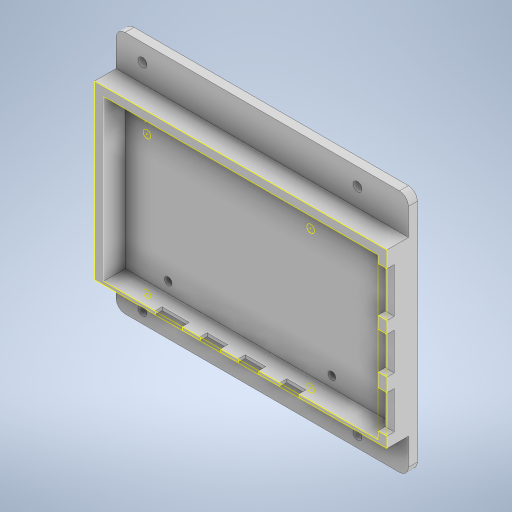
# Autodesk Inventor part: RPIcaseBottom
Saved by Autodesk Inventor 2024 (Build 280153000, 153)
## iProperties
Created: 2023-07-18
Part Number: RPIcaseBottom
Material: Generic
Document SubType Name: Modeling
Designer: 18179
Density: 1 g/cm^3
Appearance: Default
Autodesk Inventor part; units mm, degrees
ref_plane "YZ Plane" through (0, 0, 0) normal (1, 0, 0) x (0, 1, 0)
ref_plane "XZ Plane" through (0, 0, 0) normal (0, 1, 0) x (-1, 0, 0)
ref_plane "XY Plane" through (0, 0, 0) normal (0, 0, 1) x (1, 0, 0)
sketch "0" plane through (0, 0, 0) normal (0, 0, 1) x (1, 0, 0)
  line L0 (79, 0) -> (0, 0)
  arc A0 (0, 0) -> (-3, -3) centre (0, -3) ccw
  line L1 (-3, -3) -> (-3, -53)
  arc A1 (-3, -53) -> (0, -56) centre (0, -53) ccw
  line L2 (0, -56) -> (79, -56)
  arc A2 (79, -56) -> (82, -53) centre (79, -53) ccw
  line L3 (82, -53) -> (82, -3)
  arc A3 (82, -3) -> (79, 0) centre (79, -3) ccw
  circle A4 centre (0.5, -3.5) radius 1.35
  circle A5 centre (0.5, -52.5) radius 1.35
  line L4 (3.73, -49.89) -> (3.73, -57.5)
  line L5 (12.67, -57.5) -> (12.67, -49.89)
  line L6 (5.03, -57.5) -> (11.37, -57.5)
  line L7 (19.75, -50.3) -> (19.75, -57.8)
  line L8 (26.25, -57.8) -> (26.25, -50.3)
  line L9 (20.2, -57.8) -> (25.8, -57.8)
  line L10 (33.25, -50.3) -> (33.25, -57.8)
  line L11 (39.75, -57.8) -> (39.75, -50.3)
  line L12 (33.7, -57.8) -> (39.3, -57.8)
  line L13 (54, -55.9) -> (54, -58.1)
  line L14 (48, -55.9) -> (48, -58.1)
  line L15 (48.3, -58.4) -> (53.7, -58.4)
  line L16 (68.53, -53.65) -> (85, -53.65)
  line L17 (85, -53.35) -> (85, -40.65)
  line L18 (85, -40.35) -> (68.53, -40.35)
  line L19 (68.44, -22.45) -> (85, -22.45)
  line L20 (85.6, -23.75) -> (85.6, -34.25)
  line L21 (68.44, -35.55) -> (85, -35.55)
  line L22 (84.8, -2.3) -> (63.85, -2.3)
  line L23 (85, -18) -> (85, -2.5)
  line L24 (63.85, -18.2) -> (84.8, -18.2)
  circle A6 centre (58.5, -3.5) radius 1.35
  circle A7 centre (58.5, -52.5) radius 1.35
  line L25 (3.73, -57.5) -> (12.67, -57.5)
  line L26 (19.75, -57.8) -> (26.25, -57.8)
  line L27 (33.25, -57.8) -> (39.75, -57.8)
  line L28 (54, -58.1) -> (53.7, -58.4)
  line L29 (48.3, -58.4) -> (48, -58.1)
  line L30 (85, -53.65) -> (85, -40.35)
  line L31 (85, -35.55) -> (85.6, -35.55)
  line L32 (85.6, -35.55) -> (85.6, -22.45)
  line L33 (85.6, -22.45) -> (85, -22.45)
  line L34 (84.8, -18.2) -> (85, -18.2)
  line L35 (85, -18.2) -> (85, -2.3)
  line L36 (85, -2.3) -> (84.8, -2.3)
  line L37 (84.8, -2.3) -> (84.8, -18.2)
  line L38 (-3, -28) -> (-18, -28)
  line L39 (3.73, -57.5) -> (-18, -57.5)
  line L40 (-18, -57.5) -> (85.6, -57.5)
  line L41 (79, 0.3263) -> (0, 0.3263)
  line L42 (39.5, 0.3263) -> (39.5, 3.5013)
  line L43 (0, -56.3549) -> (79, -56.3549)
  line L44 (3.4071, -49.89) -> (3.4071, -57.5)
  line L45 (13.029, -49.89) -> (13.029, -57.859)
  line L46 (13.029, -57.859) -> (3.73, -57.859)
  line L47 (19.369, -50.3) -> (19.369, -58.181)
  line L48 (19.369, -58.181) -> (26.631, -58.181)
  line L49 (26.631, -58.181) -> (26.631, -50.3)
  line L50 (32.869, -50.3) -> (32.869, -58.181)
  line L51 (32.869, -58.181) -> (40.131, -58.181)
  line L52 (40.131, -58.181) -> (40.131, -50.3)
  line L53 (47.619, -55.9) -> (47.619, -58.2578)
  line L54 (47.619, -58.2578) -> (48.1422, -58.781)
  line L55 (48.1422, -58.781) -> (53.8578, -58.781)
  line L56 (53.8578, -58.781) -> (54.381, -58.2578)
  line L57 (54.381, -58.2578) -> (54.381, -55.9)
  line L58 (82.381, -53) -> (82.381, -3)
  line L59 (-3.381, -3) -> (-3.381, -53)
  line L60 (-18, -57.5) -> (39.5, -57.5)
  line L61 (39.5, -57.5) -> (39.5, 3.5013) construction
  line L62 (39.5, 3.5013) -> (-18, 3.5013)
  line L63 (-18, 3.5013) -> (-18, -57.5)
  line L64 (39.5, 3.5013) -> (85.6, 3.5013)
  line L65 (85.6, 3.5013) -> (85.6, -57.5)
  line L66 (85.6, -57.5) -> (39.5, -57.5)
  line L67 (39.5, -57.5) -> (39.5, 3.5013) construction
  line L68 (-3.381, -3) -> (0, -3)
  line L69 (0, -3) -> (0, 0.3263)
  line L70 (0, 0.3263) -> (-3.381, 0.3263)
  line L71 (-3.381, 0.3263) -> (-3.381, -3)
  line L72 (79, 0.3263) -> (82.381, 0.3263)
  line L73 (82.381, 0.3263) -> (82.381, -3)
  line L74 (82.381, -3) -> (79, -3)
  line L75 (79, -3) -> (79, 0.3263)
  line L76 (79, -56.3549) -> (82.381, -56.3549)
  line L77 (82.381, -56.3549) -> (82.381, -53)
  line L78 (82.381, -53) -> (79, -53)
  line L79 (79, -53) -> (79, -56.3549)
  line L80 (-3.381, -53) -> (0, -53)
  line L81 (0, -53) -> (0, -56.3549)
  line L82 (0, -56.3549) -> (-3.381, -56.3549)
  line L83 (-3.381, -56.3549) -> (-3.381, -53)
  line L84 (85, -53.65) -> (85.6, -53.65)
  line L85 (85.6, -53.65) -> (85.6, -40.35)
  line L86 (85.6, -40.35) -> (85, -40.35)
  line L87 (85, -40.35) -> (85, -53.65)
  line L88 (85, -18.2) -> (85.6, -18.2)
  line L89 (85.6, -18.2) -> (85.6, -2.3)
  line L90 (85.6, -2.3) -> (85, -2.3)
  line L91 (85, -2.3) -> (85, -18.2)
  line L92 (-18, -28) -> (-14.825, -28)
  line L93 (-14.825, -28) -> (-3.381, -28)
  line L94 (-3.381, -28) -> (-3.381, 0.3263)
  line L95 (-3.381, 0.3263) -> (-14.825, 0.3263)
  line L96 (-14.825, 0.3263) -> (-14.825, -28)
  line L97 (-14.825, -28) -> (-3.381, -28)
  line L98 (-3.381, -28) -> (-3.381, -56.3549)
  line L99 (-3.381, -56.3549) -> (-14.825, -56.3549)
  line L100 (-14.825, -56.3549) -> (-14.825, -28)
  point P0 (19.369, -57.5)
  point P1 (19.369, -56.3549)
  point P2 (13.029, -56.3549)
  point P3 (13.029, -57.5)
  point P4 (32.869, -57.5)
  point P5 (32.869, -56.3549)
  point P6 (26.631, -56.3549)
  point P7 (26.631, -57.5)
  point P8 (47.619, -57.5)
  point P9 (47.619, -56.3549)
  point P10 (40.131, -56.3549)
  point P11 (40.131, -57.5)
  point P12 (54.381, -56.3549)
  point P13 (54.381, -57.5)
  point P14 (82.381, -53.65)
  point P15 (82.381, -35.55)
  point P16 (82.381, -40.35)
  point P17 (82.381, -18.2)
  point P18 (82.381, -22.45)
  point P19 (82.381, -2.3)
  point P20 (3.4071, -56.3549)
  dimension "d0" = 15
  dimension "d2" = 3.175
  dimension "d3" = 0.381
  dimension "d4" = 0.381
  dimension "d5" = 0.381
  dimension "d6" = 0.381
  dimension "d7" = 0.381
  dimension "d8" = 3.175
  constraints: 202 end point, 27 parallel, 16 perpendicular, 14 horizontal, 8 centre point, 8 point on circle, 5 point on line, 2 collinear, 2 midpoint, 2 vertical, 9 other
  measures "d0" distance of L38.start L38.end
  measures "d2" distance of L42.start L42.end
  measures "d3" distance between parallel lines of L7 L47
  measures "d4" distance between parallel lines of L10 L50
  measures "d5" distance between parallel lines of L29 L54
  measures "d6" distance between parallel lines of L3 L58
  measures "d7" distance between parallel lines of L1 L59
  measures "d8" distance of L38.end L92.end
extrude "Extrusion1" add sketch "0" along normal blind 7.62 contours L41 L42 L64 L65 L90 L36 L22 L73 L72 | L70 L95 L96 L38 L63 L62 L42 L41 | L69 L68 A4 | A4 L68 L69 | L24 L34 L88 L65 L33 L19 L58 | L80 L81 A5 | A5 L81 L80 | L100 L99 L82 L43 L44 L39 L63 L38 | L21 L31 L65 L86 L18 L58 | L16 L84 L65 L40 L57 L43 L76 L77 | L43 L47 L40 L45 | L43 L50 L40 L49 | L53 L40 L52 L43 | A6 | A7
sketch "Sketch3" plane through (0, 0, 0) normal (0, 0, -1) x (-1, 0, 0)
  line L0 (-85.6, 3.5013) -> (18, 3.5013) projected
  line L1 (-54.381, -57.5) -> (-85.6, -57.5) projected
  line L2 (18, 3.5013) -> (-85.6, 3.5013)
  line L3 (-85.6, 3.5013) -> (-85.6, -57.5)
  line L4 (-85.6, -57.5) -> (18, -57.5)
  line L5 (18, -57.5) -> (18, 3.5013)
  circle A0 centre (-0.5, -3.5) radius 1.35 projected
  circle A1 centre (-0.5, -52.5) radius 1.35 projected
  circle A2 centre (-58.5, -52.5) radius 1.35 projected
  circle A3 centre (-58.5, -3.5) radius 1.35 projected
  line L6 (18, -57.5) -> (-85.6, -57.5)
  line L7 (-85.6, -57.5) -> (-85.6, -67.025)
  line L8 (-82.425, -70.2) -> (14.825, -70.2)
  line L9 (18, -67.025) -> (18, -57.5)
  line L10 (18, 3.5013) -> (-85.6, 3.5013)
  line L11 (-85.6, 3.5013) -> (-85.6, 13.0263)
  line L12 (-82.425, 16.2013) -> (14.825, 16.2013)
  line L13 (18, 13.0263) -> (18, 3.5013)
  arc A4 (18, 13.0263) -> (14.825, 16.2013) centre (14.825, 13.0263) ccw
  arc A5 (-82.425, 16.2013) -> (-85.6, 13.0263) centre (-82.425, 13.0263) ccw
  line L14 (-0.5, -52.5) -> (-58.5, -3.5) construction
  line L15 (-58.5, -3.5) -> (-58.5, -52.5) construction
  line L16 (-58.5, -52.5) -> (-0.5, -3.5) construction
  arc A6 (14.825, -70.2) -> (18, -67.025) centre (14.825, -67.025) ccw
  arc A7 (-85.6, -67.025) -> (-82.425, -70.2) centre (-82.425, -67.025) ccw
  line L17 (-29.5, -28) -> (-29.5, -66.1) construction
  line L18 (-29.5, -66.1) -> (-29.5, 10.1) construction
  line L19 (-29.5, 10.1) -> (8.6, 10.1) construction
  line L20 (8.6, 10.1) -> (-67.6, 10.1) construction
  line L21 (-29.5, -66.1) -> (8.6, -66.1) construction
  line L22 (8.6, -66.1) -> (-67.6, -66.1) construction
  circle A8 centre (8.6, -66.1) radius 1.5875
  circle A9 centre (-67.6, -66.1) radius 1.5875
  circle A10 centre (-67.6, 10.1) radius 1.5875
  circle A11 centre (8.6, 10.1) radius 1.5875
  point P0 (0, 0)
  point P1 (-85.6, -70.2)
  point P2 (-85.6, 16.2013)
  dimension "d11" = 12.7
  dimension "d12" = 12.7
  dimension "d13" = 3.175
  dimension "d14" = 3.175
  dimension "d15" = 38.1
  dimension "d16" = 76.2
  dimension "d17" = 38.1
  dimension "d18" = 76.2
  dimension "d19" = 38.1
  dimension "d20" = 76.2
  dimension "d21" = 3.175
  dimension "d22" = 3.175
  dimension "d23" = 3.175
  dimension "d24" = 3.175
  constraints: 42 end point, 8 centre point, 8 point on circle, 8 point on line, 8 tangent, 6 parallel, 5 perpendicular, 4 coincident, 3 horizontal, 2 equal radius, 2 vertical, 1 midpoint
  measures "d11" distance of point (-85.6, -70.2) L6.end
  measures "d12" distance of L10.end point (-85.6, 16.201)
  measures "d13" radius of A4
  measures "d14" radius of A6
  measures "d15" distance of L17.start L17.end
  measures "d16" distance of L17.end L18.end
  measures "d17" distance of L18.end L19.end
  measures "d18" distance of L19.end L20.end
  measures "d19" distance of L17.end L21.end
  measures "d20" distance of L21.end L22.end
  measures "d21" diameter of A8
  measures "d22" diameter of A9
  measures "d23" diameter of A10
  measures "d24" diameter of A11
extrude "Extrusion2" add sketch "Sketch3" along normal blind 3.175
sketch "Sketch4" plane through (0.5, -52.5, 7.62) normal (0, 0, 1) x (1, 0, 0)
  circle A0 centre (0, 49) radius 1.35 projected
  circle A1 centre (0, 0) radius 1.35 projected
  circle A2 centre (58, 0) radius 1.35 projected
  circle A3 centre (58, 49) radius 1.35 projected
  point P0 (-0.5, 52.5)
extrude "Extrusion3" cut sketch "Sketch4" against normal through all
sketch "Sketch6" plane through (0, 0, 0) normal (0, 0, 1) x (1, 0, 0)
  circle A0 centre (-8.6, -66.1) radius 1.5875 projected
  circle A1 centre (67.6, -66.1) radius 1.5875 projected
  circle A2 centre (58.5, -3.5) radius 1.35 projected
  circle A3 centre (58.5, -52.5) radius 1.35 projected
  circle A4 centre (0.5, -52.5) radius 1.35 projected
  circle A5 centre (0.5, -3.5) radius 1.35 projected
  line L0 (47.619, -57.5) -> (47.619, -56.3549) projected
  line L1 (40.131, -57.5) -> (47.619, -57.5) projected
  line L2 (40.131, -56.3549) -> (40.131, -57.5) projected
  line L3 (47.619, -56.3549) -> (40.131, -56.3549) projected
  line L4 (32.869, -57.5) -> (32.869, -56.3549) projected
  line L5 (26.631, -57.5) -> (32.869, -57.5) projected
  line L6 (26.631, -56.3549) -> (26.631, -57.5) projected
  line L7 (32.869, -56.3549) -> (26.631, -56.3549) projected
  line L8 (19.369, -57.5) -> (19.369, -56.3549) projected
  line L9 (13.029, -57.5) -> (19.369, -57.5) projected
  line L10 (13.029, -56.3549) -> (13.029, -57.5) projected
  line L11 (19.369, -56.3549) -> (13.029, -56.3549) projected
  line L12 (85.6, -35.55) -> (82.381, -35.55) projected
  line L13 (85.6, -22.45) -> (85.6, -35.55) projected
  line L14 (82.381, -22.45) -> (85.6, -22.45) projected
  line L15 (82.381, -18.2) -> (82.381, -22.45) projected
  line L16 (85.6, -18.2) -> (82.381, -18.2) projected
  line L17 (85.6, -2.3) -> (85.6, -18.2) projected
  line L18 (82.381, -2.3) -> (85.6, -2.3) projected
  line L19 (82.381, 0.3263) -> (82.381, -2.3) projected
  line L20 (-14.825, 0.3263) -> (82.381, 0.3263) projected
  line L21 (-14.825, -56.3549) -> (-14.825, 0.3263) projected
  line L22 (3.4071, -56.3549) -> (-14.825, -56.3549) projected
  line L23 (3.4071, -57.5) -> (3.4071, -56.3549) projected
  line L24 (-18, -57.5) -> (3.4071, -57.5) projected
  line L25 (-18, -67.025) -> (-18, -57.5) projected
  arc A6 (-18, -67.025) -> (-14.825, -70.2) centre (-14.825, -67.025) ccw projected
  line L26 (82.425, -70.2) -> (-14.825, -70.2) projected
  arc A7 (82.425, -70.2) -> (85.6, -67.025) centre (82.425, -67.025) ccw projected
  line L27 (85.6, -57.5) -> (85.6, -67.025) projected
  line L28 (54.381, -57.5) -> (85.6, -57.5) projected
  line L29 (54.381, -56.3549) -> (54.381, -57.5) projected
  line L30 (82.381, -56.3549) -> (54.381, -56.3549) projected
  line L31 (82.381, -53.65) -> (82.381, -56.3549) projected
  line L32 (85.6, -53.65) -> (82.381, -53.65) projected
  line L33 (85.6, -40.35) -> (85.6, -53.65) projected
  line L34 (82.381, -40.35) -> (85.6, -40.35) projected
  line L35 (82.381, -35.55) -> (82.381, -40.35) projected
  line L36 (3.4071, -57.5) -> (13.029, -57.5)
  line L37 (13.029, -57.5) -> (13.029, -56.3549)
  line L38 (13.029, -56.3549) -> (3.4071, -56.3549)
  line L39 (3.4071, -56.3549) -> (3.4071, -57.5)
  line L40 (19.369, -57.5) -> (26.631, -57.5)
  line L41 (26.631, -57.5) -> (26.631, -56.3549)
  line L42 (26.631, -56.3549) -> (19.369, -56.3549)
  line L43 (19.369, -56.3549) -> (19.369, -57.5)
  line L44 (32.869, -57.5) -> (40.131, -57.5)
  line L45 (40.131, -57.5) -> (40.131, -56.3549)
  line L46 (40.131, -56.3549) -> (32.869, -56.3549)
  line L47 (32.869, -56.3549) -> (32.869, -57.5)
  line L48 (47.619, -57.5) -> (54.381, -57.5)
  line L49 (54.381, -57.5) -> (54.381, -56.3549)
  line L50 (54.381, -56.3549) -> (47.619, -56.3549)
  line L51 (47.619, -56.3549) -> (47.619, -57.5)
  line L52 (85.6, -53.65) -> (82.381, -53.65)
  line L53 (82.381, -53.65) -> (82.381, -40.35)
  line L54 (82.381, -40.35) -> (85.6, -40.35)
  line L55 (85.6, -40.35) -> (85.6, -53.65)
  line L56 (82.381, -35.55) -> (85.6, -35.55)
  line L57 (85.6, -35.55) -> (85.6, -22.45)
  line L58 (85.6, -22.45) -> (82.381, -22.45)
  line L59 (82.381, -22.45) -> (82.381, -35.55)
  line L60 (85.6, -18.2) -> (82.381, -18.2)
  line L61 (82.381, -18.2) -> (82.381, -2.3)
  line L62 (82.381, -2.3) -> (85.6, -2.3)
  line L63 (85.6, -2.3) -> (85.6, -18.2)
  point P0 (0, 0)
  constraints: 56 end point, 14 parallel, 7 horizontal, 7 perpendicular
extrude "Extrusion4" add sketch "Sketch6" along normal blind 5.08 contours L0 L50 L29 L48 | L44 L4 L46 L2 | L40 L8 L42 L6 | L53 L34 L33 L32 | L36 L23 L38 L10 | L59 L14 L13 L12 | L61 L18 L17 L16
sketch "Sketch7" plane through (0, 0, 7.62) normal (0, 0, 1) x (1, 0, 0)
  line L0 (-14.825, -56.3549) -> (-14.825, 0.3263) projected
  line L1 (-14.825, 0.3263) -> (82.381, 0.3263) projected
  line L2 (82.381, 0.3263) -> (82.381, -2.3) projected
  line L3 (82.381, -2.3) -> (85.6, -2.3) projected
  line L4 (85.6, -2.3) -> (85.6, 3.5013) projected
  line L5 (85.6, 3.5013) -> (-18, 3.5013) projected
  line L6 (-18, 3.5013) -> (-18, -57.5) projected
  line L7 (-18, -57.5) -> (3.4071, -57.5) projected
  line L8 (3.4071, -57.5) -> (3.4071, -56.3549) projected
  line L9 (3.4071, -56.3549) -> (-14.825, -56.3549) projected
  line L10 (82.381, -56.3549) -> (-14.825, -56.3549) projected
  line L11 (82.381, 0.3263) -> (82.381, -56.3549) projected
  line L12 (-14.825, 0.3263) -> (82.381, 0.3263) projected
  line L13 (-14.825, -56.3549) -> (-14.825, 0.3263) projected
  circle A0 centre (58.5, -3.5) radius 1.35 projected
  circle A1 centre (58.5, -52.5) radius 1.35 projected
  circle A2 centre (0.5, -52.5) radius 1.35 projected
  circle A3 centre (0.5, -3.5) radius 1.35 projected
  line L14 (13.029, -56.3549) -> (13.029, -57.5) projected
  line L15 (13.029, -56.3549) -> (3.4071, -56.3549) projected
  line L16 (3.4071, -57.5) -> (3.4071, -56.3549) projected
  line L17 (3.4071, -57.5) -> (13.029, -57.5) projected
  line L18 (19.369, -56.3549) -> (13.029, -56.3549) projected
  line L19 (13.029, -56.3549) -> (13.029, -57.5) projected
  line L20 (13.029, -57.5) -> (19.369, -57.5) projected
  line L21 (19.369, -57.5) -> (19.369, -56.3549) projected
  line L22 (26.631, -56.3549) -> (26.631, -57.5) projected
  line L23 (26.631, -56.3549) -> (19.369, -56.3549) projected
  line L24 (19.369, -57.5) -> (19.369, -56.3549) projected
  line L25 (19.369, -57.5) -> (26.631, -57.5) projected
  line L26 (26.631, -57.5) -> (32.869, -57.5) projected
  line L27 (32.869, -56.3549) -> (26.631, -56.3549) projected
  line L28 (26.631, -56.3549) -> (26.631, -57.5) projected
  line L29 (26.631, -57.5) -> (32.869, -57.5) projected
  line L30 (32.869, -57.5) -> (32.869, -56.3549) projected
  line L31 (40.131, -56.3549) -> (40.131, -57.5) projected
  line L32 (40.131, -56.3549) -> (32.869, -56.3549) projected
  line L33 (32.869, -57.5) -> (32.869, -56.3549) projected
  line L34 (32.869, -57.5) -> (40.131, -57.5) projected
  line L35 (47.619, -56.3549) -> (40.131, -56.3549) projected
  line L36 (40.131, -56.3549) -> (40.131, -57.5) projected
  line L37 (40.131, -57.5) -> (47.619, -57.5) projected
  line L38 (47.619, -57.5) -> (47.619, -56.3549) projected
  line L39 (54.381, -56.3549) -> (54.381, -57.5) projected
  line L40 (54.381, -56.3549) -> (47.619, -56.3549) projected
  line L41 (47.619, -57.5) -> (47.619, -56.3549) projected
  line L42 (47.619, -57.5) -> (54.381, -57.5) projected
  line L43 (82.381, -56.3549) -> (54.381, -56.3549) projected
  line L44 (54.381, -56.3549) -> (54.381, -57.5) projected
  line L45 (54.381, -57.5) -> (85.6, -57.5) projected
  line L46 (85.6, -57.5) -> (85.6, -53.65) projected
  line L47 (85.6, -53.65) -> (82.381, -53.65) projected
  line L48 (82.381, -53.65) -> (82.381, -56.3549) projected
  line L49 (85.6, -53.65) -> (82.381, -53.65) projected
  line L50 (85.6, -53.65) -> (85.6, -40.35) projected
  line L51 (82.381, -40.35) -> (85.6, -40.35) projected
  line L52 (82.381, -40.35) -> (82.381, -53.65) projected
  line L53 (85.6, -35.55) -> (82.381, -35.55) projected
  line L54 (85.6, -35.55) -> (85.6, -22.45) projected
  line L55 (82.381, -22.45) -> (85.6, -22.45) projected
  line L56 (82.381, -22.45) -> (82.381, -35.55) projected
  line L57 (85.6, -18.2) -> (85.6, -2.3) projected
  line L58 (85.6, -18.2) -> (82.381, -18.2) projected
  line L59 (85.6, -18.2) -> (85.6, -2.3) projected
  line L60 (82.381, -2.3) -> (85.6, -2.3) projected
  line L61 (82.381, -2.3) -> (82.381, -18.2) projected
  line L62 (85.6, -18.2) -> (82.381, -18.2) projected
  line L63 (82.381, -18.2) -> (82.381, -22.45) projected
  line L64 (82.381, -22.45) -> (85.6, -22.45) projected
  line L65 (85.6, -22.45) -> (85.6, -18.2) projected
  line L66 (85.6, -40.35) -> (85.6, -35.55) projected
  line L67 (85.6, -35.55) -> (82.381, -35.55) projected
  line L68 (82.381, -35.55) -> (82.381, -40.35) projected
  line L69 (82.381, -40.35) -> (85.6, -40.35) projected
  point P0 (0, 0)
body "Solid1"
